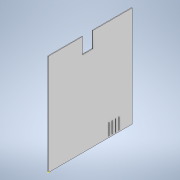
# Autodesk Inventor part: 220310 Sides
Saved by Autodesk Inventor 2022 (Build 260153000, 153)
## iProperties
Created: 2022-03-10
Part Number: 220310 Sides
Material: Generic
Document SubType Name: Modeling
Designer: josephinew
Density: 1 g/cm^3
Appearance: Default
Author: josephinew
Autodesk Inventor part; units mm, degrees
ref_plane "YZ Plane" through (0, 0, 0) normal (1, 0, 0) x (0, 1, 0)
ref_plane "XZ Plane" through (0, 0, 0) normal (0, 1, 0) x (-1, 0, 0)
ref_plane "XY Plane" through (0, 0, 0) normal (0, 0, 1) x (1, 0, 0)
sketch "Sketch1" plane through (0, 0, 0) normal (1, 0, 0) x (0, 1, 0)
  line L0 (0, 0) -> (488.95, 0)
  line L1 (488.95, -406.4) -> (0, -406.4)
  line L2 (0, -406.4) -> (0, 0)
  line L3 (488.95, 0) -> (488.95, -165.1)
  line L4 (488.95, -165.1) -> (412.75, -165.1)
  line L5 (412.75, -165.1) -> (412.75, -215.9)
  line L6 (412.75, -215.9) -> (488.95, -215.9)
  line L7 (488.95, 0) -> (488.95, -165.1)
  line L8 (488.95, -215.9) -> (488.95, -406.4)
  constraints: 18 end point, 6 perpendicular, 3 parallel, 1 horizontal
extrude "Extrusion1" add sketch "Sketch1" along normal blind 3.175
sketch "Sketch2" plane through (3.175, 0, 0) normal (1, 0, 0) x (0, 0, -1)
  line L0 (0, 0) -> (0, 488.95)
  line L1 (406.4, 488.95) -> (406.4, 0)
  line L2 (406.4, 0) -> (0, 0)
  line L3 (0, 488.95) -> (165.1, 488.95)
  line L4 (165.1, 488.95) -> (165.1, 412.75)
  line L5 (165.1, 412.75) -> (215.9, 412.75)
  line L6 (215.9, 412.75) -> (215.9, 488.95)
  line L7 (0, 488.95) -> (165.1, 488.95)
  line L8 (215.9, 488.95) -> (406.4, 488.95)
  line L9 (342.9, 63.5) -> (339.725, 63.5)
  line L10 (0, 457.2) -> (0, 0)
  line L11 (0, 3.175) -> (0, 98.425)
  line L12 (342.9, 3.175) -> (346.075, 3.175)
  line L13 (346.075, 3.175) -> (342.9, 3.175)
  line L14 (292.1, 63.5) -> (292.1, 6.35)
  line L15 (295.275, 63.5) -> (292.1, 63.5)
  line L16 (307.975, 63.5) -> (307.975, 6.35)
  line L17 (307.975, 63.5) -> (307.975, 6.35)
  line L18 (311.15, 63.5) -> (307.975, 63.5)
  line L19 (311.15, 6.35) -> (311.15, 63.5)
  line L20 (311.15, 63.5) -> (311.15, 6.35)
  line L21 (323.85, 6.35) -> (323.85, 63.5)
  line L22 (323.85, 63.5) -> (323.85, 6.35)
  line L23 (327.025, 63.5) -> (323.85, 63.5)
  line L24 (374.65, 3.175) -> (377.825, 3.175)
  line L25 (327.025, 63.5) -> (323.85, 63.5)
  line L26 (327.025, 6.35) -> (327.025, 63.5)
  line L27 (327.025, 63.5) -> (327.025, 6.35)
  line L28 (390.525, 3.175) -> (393.7, 3.175)
  line L29 (342.9, 63.5) -> (339.725, 63.5)
  line L30 (342.9, 6.35) -> (342.9, 63.5)
  line L31 (406.4, 98.425) -> (406.4, 3.175)
  line L32 (295.275, 6.35) -> (295.275, 63.5)
  line L33 (339.725, 6.35) -> (339.725, 63.5)
  line L34 (339.725, 63.5) -> (339.725, 6.35)
  line L35 (358.775, 3.175) -> (361.95, 3.175)
  line L36 (311.15, 63.5) -> (307.975, 63.5)
  line L37 (406.4, 0) -> (406.4, 3.175)
  line L38 (292.1, 6.35) -> (295.275, 6.35)
  line L39 (307.975, 6.35) -> (311.15, 6.35)
  line L40 (323.85, 6.35) -> (327.025, 6.35)
  line L41 (339.725, 6.35) -> (342.9, 6.35)
  dimension "d8" = 3.175
  constraints: 84 end point, 7 perpendicular, 4 parallel, 3 collinear, 1 point on line
  measures "d8" distance of L2.start L37.end
extrude "Extrusion2" cut sketch "Sketch2" against normal blind 25.4 contours L30 L41 L33 L9 | L15 L32 L38 L14 | L18 L19 L39 L16 | L21 L23 L26 L40
sketch "Sketch3" plane through (3.175, 0, 0) normal (1, 0, 0) x (0, 0, -1)
  point P0 (0, 0)
body "Solid1"
